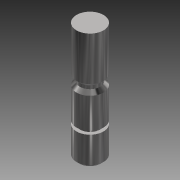
# Autodesk Inventor part: Crank shaft
Saved by Autodesk Inventor 2015 (Build 190141000, 141)
## iProperties
Created: 2008-06-06
Part Number: Crank shaft
Document SubType Name: Modeling
Designer: tangg
Density: 7.84 g/cm^3
Mass: 5.33262 g
Surface Area: 21.043 cm^2
Volume: 5.33262 cm^3
Material: Steel, High Strength Low Alloy
Appearance: Steel - Polished
Author: tangg
Autodesk Inventor part; units mm, degrees
ref_plane "YZ Plane" through (0, 0, 0) normal (1, 0, 0) x (0, 1, 0)
ref_plane "XZ Plane" through (0, 0, 0) normal (0, 1, 0) x (-1, 0, 0)
ref_plane "XY Plane" through (0, 0, 0) normal (0, 0, 1) x (1, 0, 0)
sketch "Sketch8" plane through (0, 0, 0) normal (0, 1, 0) x (-1, 0, 0)
  circle A0 centre (0, 0) radius 6.35 projected
  point P0 (0, 0)
extrude "Extrusion4" add sketch "Sketch8" against normal blind 55
chamfer "Chamfer2" distance 1.27 angle 45 1 edges at (6.35, -55, 0)
sketch "Sketch9" plane through (0, 0, 0) normal (0, 0, 1) x (1, 0, 0)
  line L0 (-6.35, 0) -> (-6.35, -53.73) projected
  line L1 (-4.7625, -22.225) -> (-4.7625, -23.8125)
  line L2 (-6.35, -25.4) -> (-6.35, -20.6375)
  line L3 (-6.35, -41.275) -> (-4.7625, -41.275)
  line L4 (-4.7625, -41.275) -> (-4.7625, -39.6875)
  line L5 (-4.7625, -39.6875) -> (-6.35, -39.6875)
  line L6 (-6.35, -39.6875) -> (-6.35, -41.275)
  line L7 (0, -64.476) -> (0, 10.746) projected
  line L8 (-4.7625, -22.225) -> (-6.35, -20.6375)
  line L9 (-4.7625, -23.8125) -> (-6.35, -25.4)
  point P0 (0, 0)
  constraints: 16 end point, 3 point on line
revolve "Revolution1" cut sketch "Sketch9" angle 360 about axis through (0, -10, 0) along (0, 1, 0)
body "Solid1"
